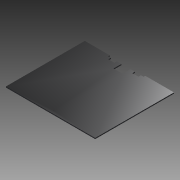
# Autodesk Inventor part: ElectronicsTopPanel
Saved by Autodesk Inventor 2015 SP1 (Build 190203100, 203)
## iProperties
Category: Panel
Created: 2015-01-14
Part Number: ElectronicsTopPanel
Material: ABS Plastic
Document SubType Name: Modeling
Designer: Jack
Density: 1.06 g/cm^3
Appearance: Smooth - Dark Gray
Mass: 810.36 g
Surface Area: 3294.73 cm^2
Volume: 764.49 cm^3
Vendor: Tap Plastics
Catalog Web Link: N/A
Author: Jack
Title: Electronics Top Panel
Autodesk Inventor part; units mm, degrees
ref_plane "YZ Plane" through (0, 0, 0) normal (1, 0, 0) x (0, 1, 0)
ref_plane "XZ Plane" through (0, 0, 0) normal (0, 1, 0) x (-1, 0, 0)
ref_plane "XY Plane" through (0, 0, 0) normal (0, 0, 1) x (1, 0, 0)
sketch "Sketch1" plane through (0, 0, 0) normal (0, 0, 1) x (1, 0, 0)
  line L0 (0, 0) -> (430, 0)
  line L1 (430, 0) -> (430, 380)
  line L2 (430, 380) -> (0, 380)
  line L3 (0, 380) -> (0, 0)
  dimension "d0" = 430
  dimension "d1" = 380
  constraints: 8 end point, 2 parallel, 1 horizontal, 1 perpendicular
  measures "d0" distance of L2.end L1.end
  measures "d1" distance of L1.end L0.end
extrude "Extrusion1" add sketch "Sketch1" along normal blind 4.7625
sketch "Sketch2" plane through (0, 0, 4.7625) normal (0, 0, 1) x (1, 0, 0)
  line L0 (0, 0) -> (430, 0) projected
  line L1 (430, 0) -> (430, 380) projected
  point P0 (213.5, 16)
  dimension "d8" = 216.5
  dimension "d33" = 16
  measures "d8" distance from line of L1 point (213.5, 16)
  measures "d33" distance from line of L0 point (213.5, 16)
hole "Hole1" at (213.5, 16, 4.7625) direction (0, 0, -1) diameter 3 end through all
sketch "Sketch4" plane through (0, 0, 4.7625) normal (0, 0, 1) x (1, 0, 0)
  line L0 (430, 0) -> (430, 380) projected
  line L1 (430, 380) -> (0, 380) projected
  line L2 (121, 380) -> (121, 372)
  line L3 (121, 372) -> (135, 372)
  line L4 (135, 372) -> (135, 360)
  line L5 (135, 360) -> (162, 360)
  line L6 (162, 360) -> (162, 372)
  line L7 (162, 372) -> (186, 372)
  line L8 (186, 372) -> (186, 334)
  line L9 (186, 334) -> (241, 334)
  line L10 (241, 334) -> (241, 372)
  line L11 (241, 372) -> (265, 372)
  line L12 (265, 372) -> (265, 360)
  line L13 (265, 360) -> (292, 360)
  line L14 (292, 360) -> (292, 372)
  line L15 (292, 372) -> (306, 372)
  line L16 (306, 372) -> (306, 380)
  dimension "d20" = 14
  dimension "d21" = 8
  dimension "d22" = 12
  dimension "d23" = 14
  dimension "d24" = 27
  dimension "d25" = 27
  dimension "d26" = 24
  dimension "d27" = 38
  dimension "d28" = 24
  dimension "d31" = 55
  dimension "d35" = 189
  constraints: 30 end point, 11 perpendicular, 8 point on line, 1 horizontal alignment, 1 vertical
  measures "d20" distance between parallel lines of L16 L14
  measures "d21" distance between parallel lines of L1 L15
  measures "d22" distance between parallel lines of L7 L5
  measures "d23" distance of L2.end L3.end
  measures "d24" distance of L4.end L5.end
  measures "d25" distance of L12.end L13.end
  measures "d26" distance between parallel lines of L12 L10
  measures "d27" distance between parallel lines of L11 L9
  measures "d28" distance between parallel lines of L6 L8
  measures "d31" distance of L8.end L9.end
  measures "d35" distance between parallel lines of L0 L10
extrude "Extrusion2" cut sketch "Sketch4" against normal up to next
body "Solid1"
